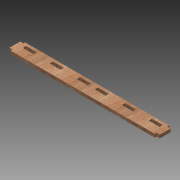
# Autodesk Inventor part: Viga delantera
Saved by Autodesk Inventor 2016 (Build 200138000, 138)
## iProperties
Created: 2016-02-08
Part Number: Viga delantera
Material: Wood (Birch)
Document SubType Name: Modeling
Designer: iberopuebla
Density: 0.55 g/cm^3
Appearance: Birch - Natural Polished
Author: iberopuebla
Autodesk Inventor part; units mm, degrees
ref_plane "YZ Plane" through (0, 0, 0) normal (1, 0, 0) x (0, 1, 0)
ref_plane "XZ Plane" through (0, 0, 0) normal (0, 1, 0) x (-1, 0, 0)
ref_plane "XY Plane" through (0, 0, 0) normal (0, 0, 1) x (1, 0, 0)
sketch "Sketch1" plane through (0, 0, 0) normal (0, 0, 1) x (1, 0, 0)
  line L0 (-30.2904, 14.2348) -> (769.7096, 14.2348)
  line L1 (769.7096, -65.7652) -> (-30.2904, -65.7652)
  line L2 (-48.2904, 4.2348) -> (-48.2904, -55.7652)
  line L3 (787.7096, 4.2348) -> (787.7096, -55.7652)
  line L4 (769.7096, 4.2348) -> (787.7096, 4.2348)
  line L5 (787.7096, -55.7652) -> (769.7096, -55.7652)
  line L6 (769.7096, 14.2348) -> (769.7096, 4.2348)
  line L7 (769.7096, -55.7652) -> (769.7096, -65.7652)
  line L8 (769.7096, -70.7652) -> (769.7096, -55.7652)
  line L9 (769.7096, 4.2348) -> (769.7096, 14.2348)
  line L10 (-48.2904, 4.2348) -> (-30.2904, 4.2348)
  line L11 (-30.2904, -55.7652) -> (-48.2904, -55.7652)
  line L12 (-30.2904, -75.7652) -> (-30.2904, -55.7652)
  line L13 (-30.2904, 4.2348) -> (-30.2904, 14.2348)
  line L14 (-30.2904, 14.2348) -> (-30.2904, 4.2348)
  line L15 (-30.2904, -55.7652) -> (-30.2904, -65.7652)
  point P0 (0, 0)
  dimension "d8" = 60
  dimension "d10" = 60
  dimension "d12" = 800
  dimension "d13" = 800
  dimension "d16" = 80
  dimension "d17" = 10
  dimension "d18" = 10
  dimension "d19" = 18
  dimension "d20" = 18
  dimension "d21" = 18
  dimension "d22" = 18
  constraints: 32 end point, 5 parallel, 4 horizontal, 2 perpendicular
  measures "d8" distance between parallel lines of L5 L4
  measures "d10" distance between parallel lines of L11 L10
  measures "d12" distance of L0.start L0.end
  measures "d13" distance of L1.start L1.end
  measures "d16" distance between parallel lines of L1 L0
  measures "d17" distance between parallel lines of L1 L11
  measures "d18" distance between parallel lines of L1 L5
  measures "d19" distance between parallel lines of L13 L2
  measures "d20" distance between parallel lines of L12 L2
  measures "d21" distance between parallel lines of L7 L3
  measures "d22" distance between parallel lines of L3 L6
extrude "Extrusion1" add sketch "Sketch1" along normal blind 18
sketch "Sketch2" plane through (0, 0, 18) normal (0, 0, 1) x (1, 0, 0)
  line L0 (-30.2904, 4.2348) -> (-31.4218, 5.3662)
  line L1 (-30.2904, 4.2348) -> (-48.2904, 4.2348) projected
  line L2 (-30.2904, -55.7652) -> (-31.4218, -56.8966)
  line L3 (769.7096, 4.2348) -> (770.841, 5.3662)
  line L4 (769.7096, -55.7652) -> (770.841, -56.8966)
  circle A0 centre (770.841, 5.3662) radius 1.6
  circle A1 centre (770.841, -56.8966) radius 1.6
  circle A2 centre (-31.4218, -56.8966) radius 1.6
  circle A3 centre (-31.4218, 5.3662) radius 1.6
  line L5 (787.7096, -55.7652) -> (787.7096, 4.2348) projected
  line L6 (-48.2904, 4.2348) -> (-48.2904, -55.7652) projected
  point P0 (0, 0)
  dimension "d23" = 1.6
  dimension "d24" = 45
  dimension "d25" = 1.6
  dimension "d26" = 1.6
  dimension "d27" = 3.2
  dimension "d28" = 3.2
  dimension "d30" = 3.2
  dimension "d31" = 3.2
  dimension "d34" = 836
  constraints: 8 end point, 4 centre point, 4 coincident, 1 parallel, 1 perpendicular
  measures "d23" distance of L0.start L0.end
  measures "d24" angle of L1 L0
  measures "d25" distance of L2.start L2.end
  measures "d26" distance of L3.start L3.end
  measures "d27" diameter of A0
  measures "d28" diameter of A1
  measures "d30" diameter of A2
  measures "d31" diameter of A3
  measures "d34" distance between parallel lines of L5 L6
extrude "Extrusion2" cut sketch "Sketch2" against normal blind 30
sketch "Sketch3" plane through (0, 0, 18) normal (0, 0, 1) x (1, 0, 0)
  line L0 (-30.2904, -0.7652) -> (769.7096, -0.7652)
  line L1 (769.7096, -0.7652) -> (769.7096, -18.7652)
  line L2 (769.7096, -18.7652) -> (-30.2904, -18.7652)
  line L3 (-30.2904, -18.7652) -> (-30.2904, -0.7652)
  line L4 (769.7096, 14.2348) -> (-30.2904, 14.2348) projected
  line L5 (769.7096, 6.4975) -> (769.7096, 14.2348) projected
  line L6 (69.7096, -0.7652) -> (69.7096, -18.7652)
  line L7 (-10.2904, -0.7652) -> (-10.2904, -18.7652)
  line L8 (49.7096, -0.7652) -> (49.7096, -18.7652)
  line L9 (689.7096, -0.7652) -> (689.7096, -18.7652)
  line L10 (749.7096, -0.7652) -> (749.7096, -18.7652)
  line L11 (669.7096, -0.7652) -> (669.7096, -18.7652)
  line L12 (119.7096, -18.7652) -> (119.7096, -0.7652)
  line L13 (139.7096, -0.7652) -> (139.7096, -18.7652)
  line L14 (199.7096, -0.7652) -> (199.7096, -18.7652)
  line L15 (619.7096, -0.7652) -> (619.7096, -18.7652)
  line L16 (219.7096, -0.7652) -> (219.7096, -18.7652)
  line L17 (269.7096, -0.7652) -> (269.7096, -18.7652)
  line L18 (519.7096, -0.7652) -> (519.7096, -18.7652)
  line L19 (539.7096, -0.7652) -> (539.7096, -18.7652)
  line L20 (599.7096, -0.7652) -> (599.7096, -18.7652)
  line L21 (469.7096, -0.7652) -> (469.7096, -18.7652)
  line L22 (369.7096, -0.7652) -> (369.7096, -18.7652)
  line L23 (289.7096, -0.7652) -> (289.7096, -18.7652)
  line L24 (349.7096, -0.7652) -> (349.7096, -18.7652)
  line L25 (389.7096, -0.7652) -> (389.7096, -18.7652)
  line L26 (449.7096, -0.7652) -> (449.7096, -18.7652)
  point P0 (0, 0)
  dimension "d35" = 800
  dimension "d36" = 18
  dimension "d37" = 15
  dimension "d38" = 0
  dimension "d39" = 100
  dimension "d40" = 20
  dimension "d41" = 60
  dimension "d42" = 100
  dimension "d43" = 60
  dimension "d44" = 20
  dimension "d45" = 600
  dimension "d47" = 50
  dimension "d48" = 50
  dimension "d49" = 100
  dimension "d50" = 60
  dimension "d51" = 20
  dimension "d52" = 50
  dimension "d53" = 100
  dimension "d54" = 60
  dimension "d55" = 20
  dimension "d56" = 50
  dimension "d57" = 100
  dimension "d58" = 60
  dimension "d59" = 20
  dimension "d60" = 60
  dimension "d61" = 20
  constraints: 46 end point, 22 vertical, 1 parallel, 48 other
  measures "d35" distance of L1.end L3.start
  measures "d36" distance of L1.start L1.end
  measures "d38" distance between parallel lines of L1 L5
  measures "d39" distance between parallel lines of L3 L6
  measures "d40" distance between parallel lines of L3 L7
  measures "d41" distance between parallel lines of L8 L7
  measures "d42" distance between parallel lines of L11 L1
  measures "d43" distance between parallel lines of L10 L9
  measures "d44" distance between parallel lines of L11 L9
  measures "d45" distance between parallel lines of L11 L6
  measures "d47" distance between parallel lines of L12 L6
  measures "d48" distance between parallel lines of L15 L11
  measures "d49" distance between parallel lines of L12 L16
  measures "d50" distance from line of L14 L13.start
  measures "d51" distance between parallel lines of L12 L13
  measures "d52" distance between parallel lines of L16 L17
  measures "d53" distance between parallel lines of L15 L18
  measures "d54" distance between parallel lines of L20 L19
  measures "d55" distance between parallel lines of L18 L19
  measures "d56" distance between parallel lines of L18 L21
  measures "d57" distance between parallel lines of L17 L22
  measures "d58" distance between parallel lines of L23 L24
  measures "d59" distance between parallel lines of L17 L23
  measures "d60" distance between parallel lines of L26 L25
  measures "d61" distance between parallel lines of L25 L22
extrude "Extrusion3" cut sketch "Sketch3" against normal blind 20 contours L0 L8 L2 L7 | L0 L14 L2 L13 | L0 L24 L2 L23 | L0 L26 L2 L25 | L0 L20 L2 L19 | L0 L10 L2 L9
sketch "Sketch4" plane through (0, 0, 18) normal (0, 0, 1) x (1, 0, 0)
  line L0 (-10.2904, -0.7652) -> (-9.159, -1.8966)
  line L1 (-10.2904, -0.7652) -> (-8.6904, -0.7652) construction
  line L2 (-10.2904, -18.7652) -> (-9.159, -17.6338)
  line L3 (49.7096, -18.7652) -> (48.5782, -17.6338)
  line L4 (49.7096, -0.7652) -> (48.5782, -1.8966)
  line L5 (139.7096, -0.7652) -> (140.841, -1.8966)
  line L6 (139.7096, -18.7652) -> (140.841, -17.6338)
  line L7 (199.7096, -0.7652) -> (198.5782, -1.8966)
  line L8 (199.7096, -18.7652) -> (198.5782, -17.6338)
  line L9 (289.7096, -18.7652) -> (290.841, -17.6338)
  line L10 (289.7096, -18.7652) -> (291.3096, -18.7652) construction
  line L11 (289.7096, -0.7652) -> (290.841, -1.8966)
  line L12 (349.7096, -0.7652) -> (348.5782, -1.8966)
  line L13 (349.7096, -18.7652) -> (348.5782, -17.6338)
  line L14 (389.7096, -0.7652) -> (390.841, -1.8966)
  line L15 (389.7096, -18.7652) -> (390.841, -17.6338)
  line L16 (449.7096, -0.7652) -> (448.5782, -1.8966)
  line L17 (449.7096, -18.7652) -> (448.5782, -17.6338)
  line L18 (539.7096, -0.7652) -> (540.841, -1.8966)
  line L19 (539.7096, -18.7652) -> (540.841, -17.6338)
  line L20 (599.7096, -0.7652) -> (598.5782, -1.8966)
  line L21 (599.7096, -18.7652) -> (598.5782, -17.6338)
  line L22 (689.7096, -0.7652) -> (690.841, -1.8966)
  line L23 (689.7096, -18.7652) -> (690.841, -17.6338)
  line L24 (749.7096, -0.7652) -> (748.5782, -1.8966)
  line L25 (749.7096, -18.7652) -> (748.5782, -17.6338)
  circle A0 centre (690.841, -1.8966) radius 1.6
  circle A1 centre (690.841, -17.6338) radius 1.6
  circle A2 centre (748.5782, -1.8966) radius 1.6
  circle A3 centre (748.5782, -17.6338) radius 1.6
  circle A4 centre (598.5782, -1.8966) radius 1.6
  circle A5 centre (598.5782, -17.6338) radius 1.6
  circle A6 centre (540.841, -1.8966) radius 1.6
  circle A7 centre (540.841, -17.6338) radius 1.6
  circle A8 centre (448.5782, -1.8966) radius 1.6
  circle A9 centre (448.5782, -17.6338) radius 1.6
  circle A10 centre (390.841, -1.8966) radius 1.6
  circle A11 centre (390.841, -17.6338) radius 1.6
  circle A12 centre (348.5782, -1.8966) radius 1.6
  circle A13 centre (348.5782, -17.6338) radius 1.6
  circle A14 centre (290.841, -1.8966) radius 1.6
  circle A15 centre (290.841, -17.6338) radius 1.6
  circle A16 centre (198.5782, -1.8966) radius 1.6
  circle A17 centre (198.5782, -17.6338) radius 1.6
  circle A18 centre (140.841, -1.8966) radius 1.6
  circle A19 centre (140.841, -17.6338) radius 1.6
  circle A20 centre (48.5782, -1.8966) radius 1.6
  circle A21 centre (48.5782, -17.6338) radius 1.6
  circle A22 centre (-9.159, -1.8966) radius 1.6
  circle A23 centre (-9.159, -17.6338) radius 1.6
  point P0 (0, 0)
  dimension "d64" = 1.6
  dimension "d65" = 45
  dimension "d66" = 1.6
  dimension "d67" = 45
  dimension "d68" = 3.2
  dimension "d69" = 3.2
  dimension "d70" = 3.2
  dimension "d71" = 3.2
  dimension "d72" = 3.2
  dimension "d73" = 3.2
  dimension "d74" = 3.2
  dimension "d75" = 3.2
  dimension "d76" = 3.2
  dimension "d77" = 3.2
  dimension "d78" = 3.2
  dimension "d79" = 3.2
  dimension "d80" = 3.2
  dimension "d81" = 3.2
  dimension "d82" = 3.2
  dimension "d83" = 3.2
  dimension "d84" = 3.2
  dimension "d85" = 3.2
  dimension "d86" = 3.2
  dimension "d87" = 3.2
  dimension "d88" = 3.2
  dimension "d89" = 3.2
  dimension "d90" = 3.2
  dimension "d91" = 3.2
  constraints: 52 end point, 24 centre point, 22 coincident, 15 perpendicular, 7 parallel, 2 equal length, 2 horizontal, 2 point on line
  measures "d64" distance of L0.start L0.end
  measures "d65" angle of L0 L1
  measures "d66" distance of L9.start L9.end
  measures "d67" angle of L10 L9
  measures "d68" diameter of A0
  measures "d69" diameter of A1
  measures "d70" diameter of A2
  measures "d71" diameter of A3
  measures "d72" diameter of A4
  measures "d73" diameter of A5
  measures "d74" diameter of A6
  measures "d75" diameter of A7
  measures "d76" diameter of A8
  measures "d77" diameter of A9
  measures "d78" diameter of A10
  measures "d79" diameter of A11
  measures "d80" diameter of A12
  measures "d81" diameter of A13
  measures "d82" diameter of A14
  measures "d83" diameter of A15
  measures "d84" diameter of A16
  measures "d85" diameter of A17
  measures "d86" diameter of A18
  measures "d87" diameter of A19
  measures "d88" diameter of A20
  measures "d89" diameter of A21
  measures "d90" diameter of A22
  measures "d91" diameter of A23
extrude "Extrusion4" cut sketch "Sketch4" against normal blind 20
body "Solid1"
